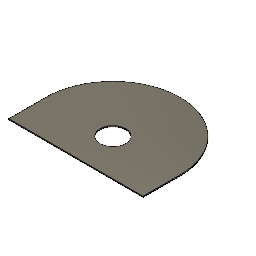
new-side-panels v2 (Autodesk Fusion 360 design; units mm, degrees)
Autodesk Fusion 360 part; units mm, degrees
note: some values were not read from the file. Set by a fixed rule: which sketch regions a step uses.
sketch "Sketch1" plane through (0, 0, 0) normal (0, 1, 0) x (1, 0, 0)
  circle A0 centre (0, 0) radius 11
  circle A1 centre (0, 0) radius 16
  line L0 (0, 0) -> (0, 19.5)
  line L1 (0, 0) -> (0, -22)
  circle A2 centre (0, 0) radius 58
  line L2 (0, -22) -> (53.6656, -22)
  line L3 (0, -22) -> (-53.6656, -22)
  line L4 (0, -22) -> (0, -26)
  line L5 (0, -26) -> (51.8459, -26)
  line L6 (0, -26) -> (-51.8459, -26)
  line L7 (0, -26) -> (0, -32)
  line L8 (0, -32) -> (48.3735, -32)
  line L9 (0, -32) -> (-48.3735, -32)
  line L10 (58, -0.0586) -> (58, -32)
  line L11 (-58, -0.0586) -> (-58, -32)
  line L12 (58, -32) -> (48.3735, -32)
  line L13 (-58, -32) -> (-48.3735, -32)
  dimension "d1" = 22
  dimension "d2" = 32
  dimension "d3" = 19.5
  dimension "d4" = 22
  dimension "d5" = 116
  dimension "d12" = 4
  dimension "d13" = 6
  constraint coincident A0.centre A1.centre
  constraint vertical L0
  constraint parallel L0 L1
  constraint coincident A2 L2.end
  constraint perpendicular L1 L2
  constraint coincident A2 L3.end
  constraint perpendicular L1 L3
  constraint perpendicular L2 L4
  constraint coincident A2 L5.end
  constraint perpendicular L4 L5
  constraint coincident A2 L6.end
  constraint perpendicular L4 L6
  constraint perpendicular L6 L7
  constraint coincident A2 L8.end
  constraint perpendicular L7 L8
  constraint coincident A2 L9.end
  constraint perpendicular L7 L9
  constraint vertical L10
  constraint coincident A2 L10.start
  constraint vertical L11
  constraint coincident A2 L11.start
  measures "d1" diameter of A0
  measures "d2" diameter of A1
  measures "d3" distance of A0.centre L0.end
  measures "d4" distance of A1.centre L1.end A0
  measures "d5" diameter of A2
  measures "d12" distance of L1.end L4.end A0
  measures "d13" distance of L4.end L7.end
extrude "Extrude1" add sketch "Sketch1" along normal blind 1 contours A0 A1 L0 L1 | A0 A1 L0 L1 | A2 L2 L3 makes body 1
sketch "Sketch2" plane through (0, 1, 0) normal (0, 1, 0) x (-1, 0, 0)
  circle A0 centre (0, 0) radius 11
  arc A1 (-53.6656, 22) -> (53.6656, 22) centre (0, 0) ccw
  line L0 (53.6656, 22) -> (-53.6656, 22)
  circle A2 centre (0, 0) radius 60.286
  line L1 (58.0702, 16.194) -> (-58.0702, 16.194)
  circle A3 centre (0, 0) radius 12.5551
  line L2 (-5.4468, 11.3121) -> (-5.4468, 16.194)
  line L3 (4.2213, 16.194) -> (4.2213, 11.8242)
  line L4 (-1.2899, -12.4887) -> (-1.2899, -60.2722)
  line L5 (2.0297, -12.39) -> (2.0297, -60.2518)
  constraint concentric A0 A2
  constraint coincident A2 L1.start
  constraint coincident A2 L1.end
  constraint parallel L0 L1
  constraint concentric A2 A3
  constraint coincident A3 L2.start
  constraint coincident L1 L2.end
  constraint perpendicular L1 L2
  constraint coincident L1 L3.start
  constraint coincident A3 L3.end
  constraint perpendicular L1 L3
  constraint coincident A3 L4.start
  constraint coincident A2 L4.end
  constraint parallel L3 L4
  constraint coincident A3 L5.start
  constraint coincident A2 L5.end
  constraint vertical L5
extrude "Extrude2" cut sketch "Sketch2" against normal blind 25 contours A1 L1 A3 L2 L4 | A1 A2 L1 L4 bodies 1
extrude "Extrude3" cut sketch "Sketch2" against normal blind 20 contours A1 A2 L1 L5 | A1 L1 A3 L3 L5 bodies 1
extrude "Extrude1'" add sketch "Sketch1" along normal blind 1 separate body contours A0 A1 L0 L1 | A0 A1 L0 L1 | A2 L2 L3 | A2 L11 L13 | A2 L10 L12 | A2 L3 L4 L6 | A2 L2 L4 L5 | A2 L6 L7 L9 | A2 L5 L7 L8 makes body 2 in component "Component"
delete_face "DeleteFace1" 1 faces at (54.7912, 0.3333, 32) on bodies 2 in component "Component"
delete_face "DeleteFace2" 1 faces at (-54.7912, 0.3333, 32) on bodies 2 in component "Component"
sketch "Sketch1 (2)" plane through (0, 1, 0) normal (0, 1, 0) x (-1, 0, 0) in component "Component"
  circle A0 centre (0, 0) radius 11
  line L0 (58, 32) -> (-58, 32)
  line L1 (-58, 32) -> (-58, 0.0586)
  arc A1 (-58, 0.0586) -> (58, 0.0586) centre (0, 0) ccw
  line L2 (58, 0.0586) -> (58, 32)
  line L3 (56, 30) -> (-56, 30)
  line L4 (-56, 30) -> (-56, 0.0576)
  arc A2 (-56, 0.0576) -> (56, 0.0576) centre (0, 0) ccw
  line L5 (56, 0.0576) -> (56, 30)
  circle A3 centre (0, 0) radius 13
  line L6 (0, -56) -> (1, -55.9911)
  line L7 (1, -55.9911) -> (-1, -55.9911)
  line L8 (-1, -55.9911) -> (-1, -12.8777)
  line L9 (-1, -12.8777) -> (1, -12.8777)
  line L10 (1, -12.8777) -> (1, -55.9911)
  line L11 (0.852, 12.9721) -> (-1.148, 12.9721)
  line L12 (-1.148, 12.9721) -> (-1.148, 30)
  line L13 (-1.148, 30) -> (0.852, 30)
  line L14 (0.852, 30) -> (0.852, 12.9721)
  line L15 (-12.8838, 1.7346) -> (-55.9806, 1.7346)
  line L16 (-55.9806, 1.7346) -> (-55.9806, -0.2654)
  line L17 (-55.9806, -0.2654) -> (-12.8838, -0.2654)
  line L18 (-12.8838, -0.2654) -> (-12.8838, 1.7346)
  line L19 (12.9159, 1.4767) -> (56, 1.4767)
  line L20 (56, 1.4767) -> (56, -0.5233)
  line L21 (56, -0.5233) -> (12.9159, -0.5233)
  line L22 (12.9159, -0.5233) -> (12.9159, 1.4767)
  dimension "d16" = -2
  dimension "d17" = 2
  dimension "d18" = 1
  dimension "d19" = 2
  dimension "d20" = 2
  dimension "d21" = 2
  dimension "d22" = 2
  constraint midpoint A2 L6.start
  constraint coincident A2 L6.end
  constraint horizontal L7
  constraint vertical L8
  constraint horizontal L9
  constraint vertical L10
  constraint horizontal L11
  constraint vertical L12
  constraint horizontal L13
  constraint vertical L14
  constraint coincident A3 L11.start
  constraint horizontal L15
  constraint vertical L16
  constraint horizontal L17
  constraint vertical L18
  constraint coincident A3 L15.start
  constraint horizontal L19
  constraint vertical L20
  constraint horizontal L21
  constraint vertical L22
  constraint coincident A3 L19.start
  measures "d18" distance of L6.start L6.end
  measures "d19" distance of L6.end L7.end
  measures "d20" distance of L11.start L11.end
  measures "d21" distance of L15.start L17.end
  measures "d22" distance of L19.start L21.end
component "Component" placed x (1, 0, 0) y (0, 1, 0) z (0, 0, 1) at (0, 0, 0)
hidden bodies 1
equation "d5 = 130 mm - 14 mm"
